Autodesk Fusion 360 part; units mm, degrees
(part 2 of 2)
sketch "gear_rotate" plane through (0, 106, 0) normal (0, 1, 0) x (-1, 0, 0) in component "blades_1"
  circle A0 centre (20, 80) radius 9.795
  circle A1 centre (20, 80) radius 17.5
  line L0 (21.5473, 97.4315) -> (21.8215, 99.4126)
  line L1 (23.9058, 97.0586) -> (23.9058, 99.0586)
  spline S0 degree 2 poles (21.8215, 99.4126) (22.2678, 101.585) (23, 102) knots 0 0 0 0.292323 0.292323 0.292323 weights 1 1.849217 1
  line L2 (23, 102) -> (23.3581, 102)
  spline S1 degree 2 poles (23.3581, 102) (23.9058, 101.7471) (23.9058, 99.0586) knots 0 0 0 0.303585 0.303585 0.303585 weights 1 0.944579 1
  line L3 (16.0849, 97.0564) -> (15.7335, 99.0253)
  spline S2 degree 2 poles (15.7335, 99.0253) (15.4867, 101.2294) (16.0548, 101.8503) knots 0 0 0 0.292323 0.292323 0.292323 weights 1 1.849217 1
  line L4 (16.0548, 101.8503) -> (16.3954, 101.961)
  spline S3 degree 2 poles (16.3954, 101.961) (16.9945, 101.8897) (17.8253, 99.3327) knots 0 0 0 0.303585 0.303585 0.303585 weights 1 0.944579 1
  line L5 (18.4433, 97.4306) -> (17.8253, 99.3327)
  line L6 (11.0058, 95.0118) -> (10.0632, 96.7757)
  spline S4 degree 2 poles (10.0632, 96.7757) (9.1473, 98.7956) (9.4958, 99.5617) knots 0 0 0 0.292323 0.292323 0.292323 weights 1 1.849217 1
  line L7 (9.4958, 99.5617) -> (9.7855, 99.7722)
  spline S5 degree 2 poles (9.7855, 99.7722) (10.3773, 99.8896) (11.9576, 97.7145) knots 0 0 0 0.303585 0.303585 0.303585 weights 1 0.944579 1
  line L8 (13.1331, 96.0965) -> (11.9576, 97.7145)
  line L9 (6.8071, 91.4977) -> (5.3655, 92.884)
  spline S6 degree 2 poles (5.3655, 92.884) (3.8703, 94.5221) (3.965, 95.3583) knots 0 0 0 0.292323 0.292323 0.292323 weights 1 1.849217 1
  line L10 (3.965, 95.3583) -> (4.1755, 95.648)
  spline S7 degree 2 poles (4.1755, 95.648) (4.702, 95.9425) (6.8771, 94.3622) knots 0 0 0 0.303585 0.303585 0.303585 weights 1 0.944579 1
  line L11 (8.4951, 93.1867) -> (6.8771, 94.3622)
  line L12 (3.8998, 86.8582) -> (2.1004, 87.7311)
  spline S8 degree 2 poles (2.1004, 87.7311) (0.1722, 88.827) (0.0038, 89.6515) knots 0 0 0 0.292323 0.292323 0.292323 weights 1 1.849217 1
  line L13 (0.0038, 89.6515) -> (0.1145, 89.9921)
  spline S9 degree 2 poles (0.1145, 89.9921) (0.5243, 90.4349) (3.0812, 89.6041) knots 0 0 0 0.303585 0.303585 0.303585 weights 1 0.944579 1
  line L14 (4.9833, 88.9861) -> (3.0812, 89.6041)
  line L15 (2.5685, 81.5473) -> (0.5874, 81.8215)
  spline S10 degree 2 poles (0.5874, 81.8215) (-1.585, 82.2678) (-2, 83) knots 0 0 0 0.292323 0.292323 0.292323 weights 1 1.849217 1
  line L16 (-2, 83) -> (-2, 83.3581)
  spline S11 degree 2 poles (-2, 83.3581) (-1.7471, 83.9058) (0.9414, 83.9058) knots 0 0 0 0.303585 0.303585 0.303585 weights 1 0.944579 1
  line L17 (2.9414, 83.9058) -> (0.9414, 83.9058)
  line L18 (2.9436, 76.0849) -> (0.9747, 75.7335)
  spline S12 degree 2 poles (0.9747, 75.7335) (-1.2294, 75.4867) (-1.8503, 76.0548) knots 0 0 0 0.292323 0.292323 0.292323 weights 1 1.849217 1
  line L19 (-1.8503, 76.0548) -> (-1.961, 76.3954)
  spline S13 degree 2 poles (-1.961, 76.3954) (-1.8897, 76.9945) (0.6673, 77.8253) knots 0 0 0 0.303585 0.303585 0.303585 weights 1 0.944579 1
  line L20 (2.5694, 78.4433) -> (0.6673, 77.8253)
  line L21 (4.9882, 71.0058) -> (3.2243, 70.0632)
  spline S14 degree 2 poles (3.2243, 70.0632) (1.2044, 69.1473) (0.4383, 69.4958) knots 0 0 0 0.292323 0.292323 0.292323 weights 1 1.849217 1
  line L22 (0.4383, 69.4958) -> (0.2278, 69.7855)
  spline S15 degree 2 poles (0.2278, 69.7855) (0.1104, 70.3773) (2.2855, 71.9576) knots 0 0 0 0.303585 0.303585 0.303585 weights 1 0.944579 1
  line L23 (3.9035, 73.1331) -> (2.2855, 71.9576)
  line L24 (8.5023, 66.8071) -> (7.116, 65.3655)
  spline S16 degree 2 poles (7.116, 65.3655) (5.4779, 63.8703) (4.6417, 63.965) knots 0 0 0 0.292323 0.292323 0.292323 weights 1 1.849217 1
  line L25 (4.6417, 63.965) -> (4.352, 64.1755)
  spline S17 degree 2 poles (4.352, 64.1755) (4.0575, 64.702) (5.6378, 66.8771) knots 0 0 0 0.303585 0.303585 0.303585 weights 1 0.944579 1
  line L26 (6.8133, 68.4951) -> (5.6378, 66.8771)
  line L27 (13.1418, 63.8998) -> (12.2689, 62.1004)
  spline S18 degree 2 poles (12.2689, 62.1004) (11.173, 60.1722) (10.3485, 60.0038) knots 0 0 0 0.292323 0.292323 0.292323 weights 1 1.849217 1
  line L28 (10.3485, 60.0038) -> (10.0079, 60.1145)
  spline S19 degree 2 poles (10.0079, 60.1145) (9.5651, 60.5243) (10.3959, 63.0812) knots 0 0 0 0.303585 0.303585 0.303585 weights 1 0.944579 1
  line L29 (11.0139, 64.9833) -> (10.3959, 63.0812)
  line L30 (18.4527, 62.5685) -> (18.1785, 60.5874)
  spline S20 degree 2 poles (18.1785, 60.5874) (17.7322, 58.415) (17, 58) knots 0 0 0 0.292323 0.292323 0.292323 weights 1 1.849217 1
  line L31 (17, 58) -> (16.6419, 58)
  spline S21 degree 2 poles (16.6419, 58) (16.0942, 58.2529) (16.0942, 60.9414) knots 0 0 0 0.303585 0.303585 0.303585 weights 1 0.944579 1
  line L32 (16.0942, 62.9414) -> (16.0942, 60.9414)
  line L33 (23.9151, 62.9436) -> (24.2665, 60.9747)
  spline S22 degree 2 poles (24.2665, 60.9747) (24.5133, 58.7706) (23.9452, 58.1497) knots 0 0 0 0.292323 0.292323 0.292323 weights 1 1.849217 1
  line L34 (23.9452, 58.1497) -> (23.6046, 58.039)
  spline S23 degree 2 poles (23.6046, 58.039) (23.0055, 58.1103) (22.1747, 60.6673) knots 0 0 0 0.303585 0.303585 0.303585 weights 1 0.944579 1
  line L35 (21.5567, 62.5694) -> (22.1747, 60.6673)
  line L36 (28.9942, 64.9882) -> (29.9368, 63.2243)
  spline S24 degree 2 poles (29.9368, 63.2243) (30.8527, 61.2044) (30.5042, 60.4383) knots 0 0 0 0.292323 0.292323 0.292323 weights 1 1.849217 1
  line L37 (30.5042, 60.4383) -> (30.2145, 60.2278)
  spline S25 degree 2 poles (30.2145, 60.2278) (29.6227, 60.1104) (28.0424, 62.2855) knots 0 0 0 0.303585 0.303585 0.303585 weights 1 0.944579 1
  line L38 (26.8669, 63.9035) -> (28.0424, 62.2855)
  line L39 (33.1929, 68.5023) -> (34.6345, 67.116)
  spline S26 degree 2 poles (34.6345, 67.116) (36.1297, 65.4779) (36.035, 64.6417) knots 0 0 0 0.292323 0.292323 0.292323 weights 1 1.849217 1
  line L40 (36.035, 64.6417) -> (35.8245, 64.352)
  spline S27 degree 2 poles (35.8245, 64.352) (35.298, 64.0575) (33.1229, 65.6378) knots 0 0 0 0.303585 0.303585 0.303585 weights 1 0.944579 1
  line L41 (31.5049, 66.8133) -> (33.1229, 65.6378)
  line L42 (36.1002, 73.1418) -> (37.8996, 72.2689)
  spline S28 degree 2 poles (37.8996, 72.2689) (39.8278, 71.173) (39.9962, 70.3485) knots 0 0 0 0.292323 0.292323 0.292323 weights 1 1.849217 1
  line L43 (39.9962, 70.3485) -> (39.8855, 70.0079)
  spline S29 degree 2 poles (39.8855, 70.0079) (39.4757, 69.5651) (36.9188, 70.3959) knots 0 0 0 0.303585 0.303585 0.303585 weights 1 0.944579 1
  line L44 (35.0167, 71.0139) -> (36.9188, 70.3959)
  line L45 (37.4315, 78.4527) -> (39.4126, 78.1785)
  spline S30 degree 2 poles (39.4126, 78.1785) (41.585, 77.7322) (42, 77) knots 0 0 0 0.292323 0.292323 0.292323 weights 1 1.849217 1
  line L46 (42, 77) -> (42, 76.6419)
  spline S31 degree 2 poles (42, 76.6419) (41.7471, 76.0942) (39.0586, 76.0942) knots 0 0 0 0.303585 0.303585 0.303585 weights 1 0.944579 1
  line L47 (37.0586, 76.0942) -> (39.0586, 76.0942)
  line L48 (37.0564, 83.9151) -> (39.0253, 84.2665)
  spline S32 degree 2 poles (39.0253, 84.2665) (41.2294, 84.5133) (41.8503, 83.9452) knots 0 0 0 0.292323 0.292323 0.292323 weights 1 1.849217 1
  line L49 (41.8503, 83.9452) -> (41.961, 83.6046)
  spline S33 degree 2 poles (41.961, 83.6046) (41.8897, 83.0055) (39.3327, 82.1747) knots 0 0 0 0.303585 0.303585 0.303585 weights 1 0.944579 1
  line L50 (37.4306, 81.5567) -> (39.3327, 82.1747)
  line L51 (35.0118, 88.9942) -> (36.7757, 89.9368)
  spline S34 degree 2 poles (36.7757, 89.9368) (38.7956, 90.8527) (39.5617, 90.5042) knots 0 0 0 0.292323 0.292323 0.292323 weights 1 1.849217 1
  line L52 (39.5617, 90.5042) -> (39.7722, 90.2145)
  spline S35 degree 2 poles (39.7722, 90.2145) (39.8896, 89.6227) (37.7145, 88.0424) knots 0 0 0 0.303585 0.303585 0.303585 weights 1 0.944579 1
  line L53 (36.0965, 86.8669) -> (37.7145, 88.0424)
  line L54 (31.4977, 93.1929) -> (32.884, 94.6345)
  spline S36 degree 2 poles (32.884, 94.6345) (34.5221, 96.1297) (35.3583, 96.035) knots 0 0 0 0.292323 0.292323 0.292323 weights 1 1.849217 1
  line L55 (35.3583, 96.035) -> (35.648, 95.8245)
  spline S37 degree 2 poles (35.648, 95.8245) (35.9425, 95.298) (34.3622, 93.1229) knots 0 0 0 0.303585 0.303585 0.303585 weights 1 0.944579 1
  line L56 (33.1867, 91.5049) -> (34.3622, 93.1229)
  line L57 (26.8582, 96.1002) -> (27.7311, 97.8996)
  spline S38 degree 2 poles (27.7311, 97.8996) (28.827, 99.8278) (29.6515, 99.9962) knots 0 0 0 0.292323 0.292323 0.292323 weights 1 1.849217 1
  line L58 (29.6515, 99.9962) -> (29.9921, 99.8855)
  spline S39 degree 2 poles (29.9921, 99.8855) (30.4349, 99.4757) (29.6041, 96.9188) knots 0 0 0 0.303585 0.303585 0.303585 weights 1 0.944579 1
  line L59 (28.9861, 95.0167) -> (29.6041, 96.9188)
  dimension "d83" = 35
  dimension "d84" = 2
  dimension "d85" = 2
  dimension "d87" = 360
  constraint concentric A0 A1
  constraint coincident A1 L0.start
  constraint coincident A1 L1.start
  constraint vertical L1
  constraint horizontal L2
  measures "d83" diameter of A1
  measures "d84" distance of L0.start L0.end
  measures "d85" distance of L1.start L1.end
extrude "Extrude4'''" add sketch "gear_rotate" along normal blind 10 separate body makes body 41 in component "blades_1"
move_body "Move13" bodies 41 to x (1, 0, 0) y (0, 1, 0) z (0, 0, 1) at (40, -10, 0) in component "blades_1"
move_body "Move14" bodies 28 to x (-1, 0, 0) y (0, -1, 0) z (0, 0, 1) at (40.2232, -120.0001, 0) in component "blades_1"
move_body "Move15" bodies 30 to x (-1, 0, 0) y (0, -1, 0) z (0, 0, 1) at (40.2232, -40.0001, 0) in component "blades_1"
move_body "Move16" bodies 31 to x (-1, 0, 0) y (0, -1, 0) z (0, 0, 1) at (40.2232, 39.9999, 0) in component "blades_1"
move_body "Move17" bodies 32 to x (-1, 0, 0) y (0, -1, 0) z (0, 0, 1) at (40.2232, 119.9999, 0) in component "blades_1"
sketch "connect_pin_crank" plane through (0, 115, 0) normal (0, 1, 0) x (-1, 0, 0) in component "blades_1"
  line L0 (-12.7954, 68.1639) -> (-6.1473, 80.3213)
  line L1 (-6.1473, 80.3213) -> (-13.3519, 92.1574)
  line L2 (-13.3519, 92.1574) -> (-27.2046, 91.8361)
  line L3 (-27.2046, 91.8361) -> (-33.8527, 79.6787)
  line L4 (-33.8527, 79.6787) -> (-26.6481, 67.8426)
  line L5 (-26.6481, 67.8426) -> (-12.7954, 68.1639)
  point P0 (-20, 80)
  dimension "d90" = 12
  measures "d90" distance of P0 L5
sketch "detail" plane through (0, 106, 0) normal (0, 1, 0) x (-1, 0, 0) in component "blades_1"
  circle A0 centre (-20, 80) radius 9.795
  arc A1 (-8.5023, 93.1929) -> (-11.0139, 95.0167) centre (-20, 80) ccw
  line L0 (-11.0139, 95.0167) -> (-10.3959, 96.9188)
  spline S0 degree 2 poles (-10.3959, 96.9188) (-9.5651, 99.4757) (-10.0079, 99.8855) knots -0.303585 -0.303585 -0.303585 0 0 0 weights 1 0.944579 1
  line L1 (-10.0079, 99.8855) -> (-10.3485, 99.9962)
  spline S1 degree 2 poles (-10.3485, 99.9962) (-11.173, 99.8278) (-12.2689, 97.8996) knots -0.292323 -0.292323 -0.292323 0 0 0 weights 1 1.849217 1
  line L2 (-12.2689, 97.8996) -> (-13.1418, 96.1002)
  arc A2 (-13.1418, 96.1002) -> (-16.0942, 97.0586) centre (-20, 80) ccw
  line L3 (-16.0942, 97.0586) -> (-16.0942, 99.0586)
  spline S2 degree 2 poles (-16.0942, 99.0586) (-16.0942, 101.7471) (-16.6419, 102) knots -0.303585 -0.303585 -0.303585 0 0 0 weights 1 0.944579 1
  line L4 (-16.6419, 102) -> (-17, 102)
  spline S3 degree 2 poles (-17, 102) (-17.7322, 101.585) (-18.1785, 99.4126) knots -0.292323 -0.292323 -0.292323 0 0 0 weights 1 1.849217 1
  line L5 (-18.1785, 99.4126) -> (-18.4527, 97.4315)
  arc A3 (-18.4527, 97.4315) -> (-21.5567, 97.4306) centre (-20, 80) ccw
  line L6 (-21.5567, 97.4306) -> (-22.1747, 99.3327)
  spline S4 degree 2 poles (-22.1747, 99.3327) (-23.0055, 101.8897) (-23.6046, 101.961) knots -0.303585 -0.303585 -0.303585 0 0 0 weights 1 0.944579 1
  line L7 (-23.6046, 101.961) -> (-23.9452, 101.8503)
  spline S5 degree 2 poles (-23.9452, 101.8503) (-24.5133, 101.2294) (-24.2665, 99.0253) knots -0.292323 -0.292323 -0.292323 0 0 0 weights 1 1.849217 1
  line L8 (-24.2665, 99.0253) -> (-23.9151, 97.0564)
  arc A4 (-23.9151, 97.0564) -> (-26.8669, 96.0965) centre (-20, 80) ccw
  line L9 (-26.8669, 96.0965) -> (-28.0424, 97.7145)
  spline S6 degree 2 poles (-28.0424, 97.7145) (-29.6227, 99.8896) (-30.2145, 99.7722) knots -0.303585 -0.303585 -0.303585 0 0 0 weights 1 0.944579 1
  line L10 (-30.2145, 99.7722) -> (-30.5042, 99.5617)
  spline S7 degree 2 poles (-30.5042, 99.5617) (-30.8527, 98.7956) (-29.9368, 96.7757) knots -0.292323 -0.292323 -0.292323 0 0 0 weights 1 1.849217 1
  line L11 (-29.9368, 96.7757) -> (-28.9942, 95.0118)
  arc A5 (-28.9942, 95.0118) -> (-31.5049, 93.1867) centre (-20, 80) ccw
  line L12 (-31.5049, 93.1867) -> (-33.1229, 94.3622)
  spline S8 degree 2 poles (-33.1229, 94.3622) (-35.298, 95.9425) (-35.8245, 95.648) knots -0.303585 -0.303585 -0.303585 0 0 0 weights 1 0.944579 1
  line L13 (-35.8245, 95.648) -> (-36.035, 95.3583)
  spline S9 degree 2 poles (-36.035, 95.3583) (-36.1297, 94.5221) (-34.6345, 92.884) knots -0.292323 -0.292323 -0.292323 0 0 0 weights 1 1.849217 1
  line L14 (-34.6345, 92.884) -> (-33.1929, 91.4977)
  arc A6 (-33.1929, 91.4977) -> (-35.0167, 88.9861) centre (-20, 80) ccw
  line L15 (-35.0167, 88.9861) -> (-36.9188, 89.6041)
  spline S10 degree 2 poles (-36.9188, 89.6041) (-39.4757, 90.4349) (-39.8855, 89.9921) knots -0.303585 -0.303585 -0.303585 0 0 0 weights 1 0.944579 1
  line L16 (-39.8855, 89.9921) -> (-39.9962, 89.6515)
  spline S11 degree 2 poles (-39.9962, 89.6515) (-39.8278, 88.827) (-37.8996, 87.7311) knots -0.292323 -0.292323 -0.292323 0 0 0 weights 1 1.849217 1
  line L17 (-37.8996, 87.7311) -> (-36.1002, 86.8582)
  arc A7 (-36.1002, 86.8582) -> (-37.0586, 83.9058) centre (-20, 80) ccw
  line L18 (-37.0586, 83.9058) -> (-39.0586, 83.9058)
  spline S12 degree 2 poles (-39.0586, 83.9058) (-41.7471, 83.9058) (-42, 83.3581) knots -0.303585 -0.303585 -0.303585 0 0 0 weights 1 0.944579 1
  line L19 (-42, 83.3581) -> (-42, 83)
  spline S13 degree 2 poles (-42, 83) (-41.585, 82.2678) (-39.4126, 81.8215) knots -0.292323 -0.292323 -0.292323 0 0 0 weights 1 1.849217 1
  line L20 (-39.4126, 81.8215) -> (-37.4315, 81.5473)
  arc A8 (-37.4315, 81.5473) -> (-37.4306, 78.4433) centre (-20, 80) ccw
  line L21 (-37.4306, 78.4433) -> (-39.3327, 77.8253)
  spline S14 degree 2 poles (-39.3327, 77.8253) (-41.8897, 76.9945) (-41.961, 76.3954) knots -0.303585 -0.303585 -0.303585 0 0 0 weights 1 0.944579 1
  line L22 (-41.961, 76.3954) -> (-41.8503, 76.0548)
  spline S15 degree 2 poles (-41.8503, 76.0548) (-41.2294, 75.4867) (-39.0253, 75.7335) knots -0.292323 -0.292323 -0.292323 0 0 0 weights 1 1.849217 1
  line L23 (-39.0253, 75.7335) -> (-37.0564, 76.0849)
  arc A9 (-37.0564, 76.0849) -> (-36.0965, 73.1331) centre (-20, 80) ccw
  line L24 (-36.0965, 73.1331) -> (-37.7145, 71.9576)
  spline S16 degree 2 poles (-37.7145, 71.9576) (-39.8896, 70.3773) (-39.7722, 69.7855) knots -0.303585 -0.303585 -0.303585 0 0 0 weights 1 0.944579 1
  line L25 (-39.7722, 69.7855) -> (-39.5617, 69.4958)
  spline S17 degree 2 poles (-39.5617, 69.4958) (-38.7956, 69.1473) (-36.7757, 70.0632) knots -0.292323 -0.292323 -0.292323 0 0 0 weights 1 1.849217 1
  line L26 (-36.7757, 70.0632) -> (-35.0118, 71.0058)
  arc A10 (-35.0118, 71.0058) -> (-33.1867, 68.4951) centre (-20, 80) ccw
  line L27 (-33.1867, 68.4951) -> (-34.3622, 66.8771)
  spline S18 degree 2 poles (-34.3622, 66.8771) (-35.9425, 64.702) (-35.648, 64.1755) knots -0.303585 -0.303585 -0.303585 0 0 0 weights 1 0.944579 1
  line L28 (-35.648, 64.1755) -> (-35.3583, 63.965)
  spline S19 degree 2 poles (-35.3583, 63.965) (-34.5221, 63.8703) (-32.884, 65.3655) knots -0.292323 -0.292323 -0.292323 0 0 0 weights 1 1.849217 1
  line L29 (-32.884, 65.3655) -> (-31.4977, 66.8071)
  arc A11 (-31.4977, 66.8071) -> (-28.9861, 64.9833) centre (-20, 80) ccw
  line L30 (-28.9861, 64.9833) -> (-29.6041, 63.0812)
  spline S20 degree 2 poles (-29.6041, 63.0812) (-30.4349, 60.5243) (-29.9921, 60.1145) knots -0.303585 -0.303585 -0.303585 0 0 0 weights 1 0.944579 1
  line L31 (-29.9921, 60.1145) -> (-29.6515, 60.0038)
  spline S21 degree 2 poles (-29.6515, 60.0038) (-28.827, 60.1722) (-27.7311, 62.1004) knots -0.292323 -0.292323 -0.292323 0 0 0 weights 1 1.849217 1
  line L32 (-27.7311, 62.1004) -> (-26.8582, 63.8998)
  arc A12 (-26.8582, 63.8998) -> (-23.9058, 62.9414) centre (-20, 80) ccw
  line L33 (-23.9058, 62.9414) -> (-23.9058, 60.9414)
  spline S22 degree 2 poles (-23.9058, 60.9414) (-23.9058, 58.2529) (-23.3581, 58) knots -0.303585 -0.303585 -0.303585 0 0 0 weights 1 0.944579 1
  line L34 (-23.3581, 58) -> (-23, 58)
  spline S23 degree 2 poles (-23, 58) (-22.2678, 58.415) (-21.8215, 60.5874) knots -0.292323 -0.292323 -0.292323 0 0 0 weights 1 1.849217 1
  line L35 (-21.8215, 60.5874) -> (-21.5473, 62.5685)
  arc A13 (-21.5473, 62.5685) -> (-18.4433, 62.5694) centre (-20, 80) ccw
  line L36 (-18.4433, 62.5694) -> (-17.8253, 60.6673)
  spline S24 degree 2 poles (-17.8253, 60.6673) (-16.9945, 58.1103) (-16.3954, 58.039) knots -0.303585 -0.303585 -0.303585 0 0 0 weights 1 0.944579 1
  line L37 (-16.3954, 58.039) -> (-16.0548, 58.1497)
  spline S25 degree 2 poles (-16.0548, 58.1497) (-15.4867, 58.7706) (-15.7335, 60.9747) knots -0.292323 -0.292323 -0.292323 0 0 0 weights 1 1.849217 1
  line L38 (-15.7335, 60.9747) -> (-16.0849, 62.9436)
  arc A14 (-16.0849, 62.9436) -> (-13.1331, 63.9035) centre (-20, 80) ccw
  line L39 (-13.1331, 63.9035) -> (-11.9576, 62.2855)
  spline S26 degree 2 poles (-11.9576, 62.2855) (-10.3773, 60.1104) (-9.7855, 60.2278) knots -0.303585 -0.303585 -0.303585 0 0 0 weights 1 0.944579 1
  line L40 (-9.7855, 60.2278) -> (-9.4958, 60.4383)
  spline S27 degree 2 poles (-9.4958, 60.4383) (-9.1473, 61.2044) (-10.0632, 63.2243) knots -0.292323 -0.292323 -0.292323 0 0 0 weights 1 1.849217 1
  line L41 (-10.0632, 63.2243) -> (-11.0058, 64.9882)
  arc A15 (-11.0058, 64.9882) -> (-8.4951, 66.8133) centre (-20, 80) ccw
  line L42 (-8.4951, 66.8133) -> (-6.8771, 65.6378)
  spline S28 degree 2 poles (-6.8771, 65.6378) (-4.702, 64.0575) (-4.1755, 64.352) knots -0.303585 -0.303585 -0.303585 0 0 0 weights 1 0.944579 1
  line L43 (-4.1755, 64.352) -> (-3.965, 64.6417)
  spline S29 degree 2 poles (-3.965, 64.6417) (-3.8703, 65.4779) (-5.3655, 67.116) knots -0.292323 -0.292323 -0.292323 0 0 0 weights 1 1.849217 1
  line L44 (-5.3655, 67.116) -> (-6.8071, 68.5023)
  arc A16 (-6.8071, 68.5023) -> (-4.9833, 71.0139) centre (-20, 80) ccw
  line L45 (-4.9833, 71.0139) -> (-3.0812, 70.3959)
  spline S30 degree 2 poles (-3.0812, 70.3959) (-0.5243, 69.5651) (-0.1145, 70.0079) knots -0.303585 -0.303585 -0.303585 0 0 0 weights 1 0.944579 1
  line L46 (-0.1145, 70.0079) -> (-0.0038, 70.3485)
  spline S31 degree 2 poles (-0.0038, 70.3485) (-0.1722, 71.173) (-2.1004, 72.2689) knots -0.292323 -0.292323 -0.292323 0 0 0 weights 1 1.849217 1
  line L47 (-2.1004, 72.2689) -> (-3.8998, 73.1418)
  arc A17 (-3.8998, 73.1418) -> (-2.9414, 76.0942) centre (-20, 80) ccw
  line L48 (-2.9414, 76.0942) -> (-0.9414, 76.0942)
  spline S32 degree 2 poles (-0.9414, 76.0942) (1.7471, 76.0942) (2, 76.6419) knots -0.303585 -0.303585 -0.303585 0 0 0 weights 1 0.944579 1
  line L49 (2, 76.6419) -> (2, 77)
  spline S33 degree 2 poles (2, 77) (1.585, 77.7322) (-0.5874, 78.1785) knots -0.292323 -0.292323 -0.292323 0 0 0 weights 1 1.849217 1
  line L50 (-0.5874, 78.1785) -> (-2.5685, 78.4527)
  arc A18 (-2.5685, 78.4527) -> (-2.5694, 81.5567) centre (-20, 80) ccw
  line L51 (-2.5694, 81.5567) -> (-0.6673, 82.1747)
  spline S34 degree 2 poles (-0.6673, 82.1747) (1.8897, 83.0055) (1.961, 83.6046) knots -0.303585 -0.303585 -0.303585 0 0 0 weights 1 0.944579 1
  line L52 (1.961, 83.6046) -> (1.8503, 83.9452)
  spline S35 degree 2 poles (1.8503, 83.9452) (1.2294, 84.5133) (-0.9747, 84.2665) knots -0.292323 -0.292323 -0.292323 0 0 0 weights 1 1.849217 1
  line L53 (-0.9747, 84.2665) -> (-2.9436, 83.9151)
  arc A19 (-2.9436, 83.9151) -> (-3.9035, 86.8669) centre (-20, 80) ccw
  line L54 (-3.9035, 86.8669) -> (-2.2855, 88.0424)
  spline S36 degree 2 poles (-2.2855, 88.0424) (-0.1104, 89.6227) (-0.2278, 90.2145) knots -0.303585 -0.303585 -0.303585 0 0 0 weights 1 0.944579 1
  line L55 (-0.2278, 90.2145) -> (-0.4383, 90.5042)
  spline S37 degree 2 poles (-0.4383, 90.5042) (-1.2044, 90.8527) (-3.2243, 89.9368) knots -0.292323 -0.292323 -0.292323 0 0 0 weights 1 1.849217 1
  line L56 (-3.2243, 89.9368) -> (-4.9882, 88.9942)
  arc A20 (-4.9882, 88.9942) -> (-6.8133, 91.5049) centre (-20, 80) ccw
  line L57 (-6.8133, 91.5049) -> (-5.6378, 93.1229)
  spline S38 degree 2 poles (-5.6378, 93.1229) (-4.0575, 95.298) (-4.352, 95.8245) knots -0.303585 -0.303585 -0.303585 0 0 0 weights 1 0.944579 1
  line L58 (-4.352, 95.8245) -> (-4.6417, 96.035)
  spline S39 degree 2 poles (-4.6417, 96.035) (-5.4779, 96.1297) (-7.116, 94.6345) knots -0.292323 -0.292323 -0.292323 0 0 0 weights 1 1.849217 1
  line L59 (-7.116, 94.6345) -> (-8.5023, 93.1929)
  circle A21 centre (-20, 80) radius 14.8615
  constraint concentric A0 A21
extrude "Extrude5''" add sketch "connect_pin_crank" against normal blind 8 bodies 29 in component "blades_1"
extrude "Extrude6" add sketch "detail" along normal blind 2 contours A21 bodies 41 in component "blades_1"
sketch "connect_crank-pin" plane through (0, 116.1453, 0) normal (0, 1, 0) x (-1, 0, 0) in component "crank_1"
  line L0 (-22.8585, 64.732) -> (-9.0058, 65.0532)
  line L1 (-9.0058, 65.0532) -> (-2.3577, 77.2106)
  line L2 (-2.3577, 77.2106) -> (-9.5622, 89.0468)
  line L3 (-9.5622, 89.0468) -> (-23.4149, 88.7255)
  line L4 (-23.4149, 88.7255) -> (-30.063, 76.5681)
  line L5 (-30.063, 76.5681) -> (-22.8585, 64.732)
  line L6 (-2.1268, 77.216) -> (-8.8857, 64.856)
  line L7 (-8.8857, 64.856) -> (-22.9692, 64.5294)
  line L8 (-22.9692, 64.5294) -> (-30.2938, 76.5628)
  line L9 (-30.2938, 76.5628) -> (-23.5349, 88.9227)
  line L10 (-23.5349, 88.9227) -> (-9.4514, 89.2493)
  line L11 (-9.4514, 89.2493) -> (-2.1268, 77.216)
  circle A0 centre (-16.4932, 75.8529) radius 15.3386
extrude "Extrude1''''''" add sketch "connect_crank-pin" against normal blind 7 separate body contours A0 makes body 42 in component "crank_1"
sketch "handle_sketch (2)" plane through (0, 0, 0) normal (0, 1, 0) x (1, 0, 0) in component "crank_1"
  circle A0 centre (16.5, -75.85) radius 15.3158
  line L0 (29.7013, -68.0847) -> (3.2987, -68.0847)
  spline S0 degree 2 poles (29.7013, -68.0847) (23, -40) (17, -40) knots 0 0 0 3.24759 3.24759 3.24759 weights 1 3 1
  spline S1 degree 2 poles (17, -40) (11, -40) (3.2987, -68.0847) knots 0 0 0 3.282575 3.282575 3.282575 weights 1 3 1
  spline S2 degree 2 poles (3.1745, -68.3) (-17.797, -88.1458) (-14.797, -93.342) knots 0 0 0 3.24759 3.24759 3.24759 weights 1 3 1
  spline S3 degree 2 poles (-14.797, -93.342) (-11.797, -98.5381) (16.3757, -91.1653) knots 0 0 0 3.282575 3.282575 3.282575 weights 1 3 1
  circle A1 centre (16.5, -75.85) radius 15.3158
  spline S4 degree 2 poles (16.6243, -91.1653) (44.297, -99.4042) (47.297, -94.208) knots 0 0 0 3.24759 3.24759 3.24759 weights 1 3 1
  spline S5 degree 2 poles (47.297, -94.208) (50.297, -89.0119) (29.8255, -68.3) knots 0 0 0 3.282575 3.282575 3.282575 weights 1 3 1
  circle A2 centre (16.5, -75.85) radius 15.3158
  dimension "d99" = 360
  constraint coincident A0 L0.start
  constraint coincident A0 L0.end
  constraint horizontal L0
extrude "Extrude2''''" add sketch "handle_sketch (2)" along normal blind 6 separate body contours A0 A1 S4 S5 A2 | A0 S0 S1 A1 A2 | A0 S2 S3 A1 A2 makes body 43 at (38.0301, 0, 88.039) makes body 44 at (16.1704, 0, 51.4897) makes body 45 at (-4.8268, 0, 88.4024) in component "crank_1"
move_body "Move1'''" bodies 45 44 43 to x (1, 0, 0) y (0, 1, 0) z (0, 0, 1) at (0, 109, 0) in component "crank_1"
combine "Combine1''" operation add target body 42 tool bodies 43 44 45 in component "crank_1"
sketch "handle_movement" plane through (0, 115, 0) normal (0, 1, 0) x (-1, 0, 0) in component "crank_1"
  arc A0 (-16.7077, 91.1901) -> (-29.867, 68.3419) centre (-16.4932, 75.8529) ccw
  spline S0 degree 2 poles (-16.7077, 91.1901) (-44.2975, 99.4033) (-47.297, 94.208) knots 0.001635 0.001635 0.001635 3.24759 3.24759 3.24759 weights 1.002013 2.998993 1
  spline S1 degree 2 poles (-47.297, 94.208) (-50.2967, 89.0124) (-29.867, 68.3419) knots 0 0 0 3.281466 3.281466 3.281466 weights 1 2.999324 1.001351
  circle A1 centre (-40, 90) radius 3.4
  circle A2 centre (-16.9915, 48.4219) radius 3.4
  circle A3 centre (7.5119, 89.1369) radius 3.4
  dimension "d102" = 6.8
  dimension "d104" = 360
  measures "d102" diameter of A1
extrude "Extrude3''''" add sketch "handle_movement" along normal blind 25 separate body contours A1 | A2 | A3 makes body 46 at (-10.7069, 131.6667, 87.974) makes body 47 at (13.6084, 123.3333, 48.0834) makes body 48 at (42.374, 131.6667, 87.5661) in component "crank_1"
sketch "detail_1" plane through (0, 140, 0) normal (0, 1, 0) x (-1, 0, 0) in component "crank_1"
  circle A0 centre (-40, 90) radius 3.4
  circle A1 centre (-40, 90) radius 1
  constraint concentric A0 A1
sketch "detail_2" plane through (0, 140, 0) normal (0, 1, 0) x (-1, 0, 0) in component "crank_1"
  circle A0 centre (7.5119, 89.1369) radius 3.4
  circle A1 centre (7.5119, 89.1369) radius 1
  dimension "d107" = 2
  constraint concentric A0 A1
  measures "d107" diameter of A1
sketch "detail_3" plane through (0, 140, 0) normal (0, 1, 0) x (-1, 0, 0) in component "crank_1"
  circle A0 centre (-16.9915, 48.4219) radius 3.4
  circle A1 centre (-16.9915, 48.4219) radius 1
  dimension "d108" = 2
  constraint concentric A0 A1
  measures "d108" diameter of A1
extrude "Extrude4''''" cut sketch "detail_3" sketch "detail_1" sketch "detail_2" against normal blind 10 contours A1 of sketch 2 contours A1 of sketch 3 contours A1 bodies 46 47 48 in component "crank_1"
move_face "OffsetFaces1" offset 5 1 faces at (17.784, 115, 84.0525) on bodies 29 in component "blades_1"
component "holder_" placed x (1, 0, 0) y (0, 1, 0) z (0, 0, 1) at (0, 0, 0)
component "shredder_upperbody" placed x (1, 0, 0) y (0, 1, 0) z (0, 0, 1) at (0, 0, 0)
component "shredder_lowerbody" placed x (1, 0, 0) y (0, 1, 0) z (0, 0, 1) at (0, 0, 0)
component "blades_1" placed x (1, 0, 0) y (0, 1, 0) z (0, 0, 1) at (0, 0, 0)
component "blades_2" placed x (1, 0, 0) y (0, 1, 0) z (0, 0, 1) at (0, 0, 0)
component "crank_1" placed x (1, 0, 0) y (0, 1, 0) z (0, 0, 1) at (3.7897, -1.1453, 3.1106)
component "feeding_port" placed x (1, 0, 0) y (0, 1, 0) z (0, 0, 1) at (0, 0, 0)
component "optional_roof" placed x (1, 0, 0) y (0, 1, 0) z (0, 0, 1) at (0, 0, 0)
component "trashbin_removeable" placed x (1, 0, 0) y (0, 1, 0) z (0, 0, 1) at (0, 0, 0)
component "decoration" placed x (1, 0, 0) y (0, 1, 0) z (0, 0, 1) at (0, 0, 0) in component "holder_"
named bodies: "holder", "glass1", "glass2", "trashbin", "handle", "wall", "pin", "1_blade", "2_blade", "3_blade", "4_blade", "blade_replace1", "blade_replace2", "blade_replace1 (1)", "blade_replace3", "blade_replace1 (1) (1)", "blade_replace4", "1_blade (1)", "2_blade", "1_blade (1) (1)", "3_blade", "1_blade (1) (1) (1)", "gear", "handles"
